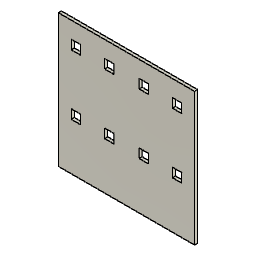
sorted_smarties_cover (Autodesk Fusion 360 design; units mm, degrees)
Autodesk Fusion 360 part; units mm, degrees
sketch "Sketch1" plane through (0, 0, 0) normal (0, 1, 0) x (1, 0, 0)
  line L0 (0, 0) -> (270, 0)
  line L1 (270, 0) -> (270, -264)
  line L2 (270, -264) -> (0, -264)
  line L3 (0, -264) -> (0, 0)
  dimension "d1" = 270
  dimension "d2" = 264
  constraint horizontal L0
  constraint vertical L1
  constraint horizontal L2
  constraint vertical L3
  constraint coincident L0.start L3.end
  measures "d1" distance of L1.end L2.end
  measures "d2" distance of L0.end L1.end
extrude "Extrude1" add sketch "Sketch1" along normal blind 6
sketch "Sketch2" plane through (0, 0, 0) normal (0, -1, 0) x (1, 0, 0)
  line L0 (270, 264) -> (0, 264)
  line L1 (0, 264) -> (0, 0)
  line L2 (0, 0) -> (270, 0)
  line L3 (270, 0) -> (270, 264)
  line L4 (25.625, 231.1665) -> (43.625, 231.1665)
  line L5 (43.625, 231.1665) -> (43.625, 213.1665)
  line L6 (43.625, 213.1665) -> (25.625, 213.1665)
  line L7 (25.625, 213.1665) -> (25.625, 231.1665)
  line L8 (91.875, 231.1665) -> (109.875, 231.1665)
  line L9 (109.875, 231.1665) -> (109.875, 213.1665)
  line L10 (109.875, 213.1665) -> (91.875, 213.1665)
  line L11 (91.875, 213.1665) -> (91.875, 231.1665)
  line L12 (160.125, 231.1665) -> (178.125, 231.1665)
  line L13 (178.125, 231.1665) -> (178.125, 213.1665)
  line L14 (178.125, 213.1665) -> (160.125, 213.1665)
  line L15 (160.125, 213.1665) -> (160.125, 231.1665)
  line L16 (226.375, 231.1665) -> (244.375, 231.1665)
  line L17 (244.375, 231.1665) -> (244.375, 213.1665)
  line L18 (244.375, 213.1665) -> (226.375, 213.1665)
  line L19 (226.375, 213.1665) -> (226.375, 231.1665)
  line L20 (25.625, 111.6665) -> (43.625, 111.6665)
  line L21 (43.625, 111.6665) -> (43.625, 93.6665)
  line L22 (43.625, 93.6665) -> (25.625, 93.6665)
  line L23 (25.625, 93.6665) -> (25.625, 111.6665)
  line L24 (91.875, 111.6665) -> (109.875, 111.6665)
  line L25 (109.875, 111.6665) -> (109.875, 93.6665)
  line L26 (109.875, 93.6665) -> (91.875, 93.6665)
  line L27 (91.875, 93.6665) -> (91.875, 111.6665)
  line L28 (160.125, 111.6665) -> (178.125, 111.6665)
  line L29 (178.125, 111.6665) -> (178.125, 93.6665)
  line L30 (178.125, 93.6665) -> (160.125, 93.6665)
  line L31 (160.125, 93.6665) -> (160.125, 111.6665)
  line L32 (226.375, 111.6665) -> (244.375, 111.6665)
  line L33 (244.375, 111.6665) -> (244.375, 93.6665)
  line L34 (244.375, 93.6665) -> (226.375, 93.6665)
  line L35 (226.375, 93.6665) -> (226.375, 111.6665)
  dimension "d5" = 18
  dimension "d6" = 18
  dimension "d7" = 18
  dimension "d8" = 18
  dimension "d9" = 18
  dimension "d10" = 18
  dimension "d11" = 270
  dimension "d12" = 264
  dimension "d13" = 25.625
  dimension "d17" = 32.8335
  dimension "d18" = 152.3335
  dimension "d19" = 48.25
  dimension "d22" = 48.25
  dimension "d24" = 25.625
  constraint horizontal L4
  constraint vertical L5
  constraint horizontal L6
  constraint vertical L7
  constraint horizontal L8
  constraint vertical L9
  constraint horizontal L10
  constraint vertical L11
  constraint horizontal L12
  constraint vertical L13
  constraint horizontal L14
  constraint vertical L15
  constraint horizontal L16
  constraint vertical L17
  constraint horizontal L18
  constraint vertical L19
  constraint collinear L12 L16
  constraint collinear L8 L12
  constraint collinear L4 L8
  constraint collinear L14 L18
  constraint collinear L10 L14
  constraint collinear L6 L10
  constraint horizontal L20
  constraint vertical L21
  constraint horizontal L22
  constraint vertical L23
  constraint horizontal L24
  constraint vertical L25
  constraint horizontal L26
  constraint vertical L27
  constraint horizontal L28
  constraint vertical L29
  constraint horizontal L30
  constraint vertical L31
  constraint horizontal L32
  constraint vertical L33
  constraint horizontal L34
  constraint vertical L35
  constraint collinear L7 L23
  constraint collinear L5 L21
  constraint collinear L11 L27
  constraint collinear L9 L25
  constraint collinear L15 L31
  constraint collinear L13 L29
  constraint collinear L19 L35
  constraint collinear L17 L33
  constraint collinear L20 L24
  constraint collinear L24 L28
  constraint collinear L28 L32
  constraint collinear L22 L26
  constraint collinear L26 L30
  constraint collinear L30 L34
  measures "d5" distance of L5.end L6.end
  measures "d6" distance of L9.end L10.end
  measures "d7" distance of L13.end L14.end
  measures "d8" distance of L17.end L18.end
  measures "d9" distance of L4.start L6.end
  measures "d10" distance of L20.start L22.end
  measures "d11" distance of L0.start L0.end
  measures "d12" distance of L0.start L2.end
  measures "d13" distance of L1 L7
  measures "d17" distance of L0 L4
  measures "d18" distance of L0 L20
  measures "d19" distance of L5 L11
  measures "d22" distance of L13 L19
  measures "d24" distance of L3 L17
extrude "Extrude2" cut sketch "Sketch2" against normal blind 6 contours L4 L5 L6 L7 | L8 L9 L10 L11 | L12 L13 L14 L15 | L16 L17 L18 L19 | L20 L21 L22 L23 | L24 L25 L26 L27 | L28 L29 L30 L31 | L32 L33 L34 L35
equation "d13 = 3 mm + ( ( 63.25 / 2 ) * 1 mm ) - ( ( 18 / 2 ) * 1 mm )"
equation "d17 = 3 mm + ( ( 77.667 / 2 ) * 1 mm ) - ( ( 18 / 2 ) * 1 mm )"
equation "d18 = 122.5 mm + ( ( 77.667 / 2 ) * 1 mm ) - ( ( 18 / 2 ) * 1 mm )"
equation "d19 = 3 mm + 63.25 mm - 18 mm"
equation "d22 = 3 mm + 63.25 mm - 18 mm"
equation "d24 = 3 mm + ( ( 63.25 / 2 ) * 1 mm ) - ( ( 18 / 2 ) * 1 mm )"
named bodies: "Sorted Smarties Cover"
